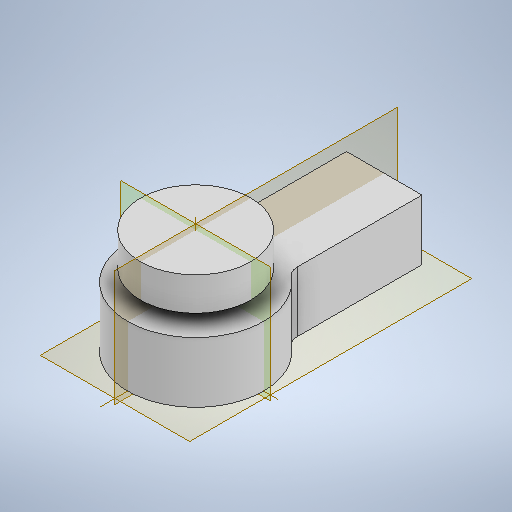
# Autodesk Inventor part: alternativeJoint2
Saved by Autodesk Inventor 2025.1 (Build 291241000, 241)
## iProperties
Created: 2024-11-07
Part Number: alternativeJoint2
Material: Generisch
Document SubType Name: Modeling
Designer: ZOMBULLI
Density: 1 g/cm^3
Appearance: Vorgabe
Author: ZOMBULLI
Autodesk Inventor part; units mm, degrees
sketch "Skizze1" plane through (0, 0, 0) normal (0, 0, 1) x (1, 0, 0)
  line L0 (5, 25) -> (-5, 25)
  line L1 (-5, 25) -> (-5, 9.3808)
  line L2 (5, 8.4853) -> (5, 25)
  arc A0 (-6.2308, 6.4944) -> (5.7273, 6.9425) centre (0, 0) ccw
  arc A1 (5, 8.4853) -> (5.7273, 6.9425) centre (7, 8.4853) ccw
  arc A2 (-6.2308, 6.4944) -> (-5, 9.3808) centre (-9, 9.3808) ccw
  line L3 (0, -25.0931) -> (0, 22.9698)
  line L4 (0, 35.0186) -> (0, -35.1118) projected
  point P0 (0, 0)
  point P1 (0, 0)
  point P2 (-5, 7.4833)
  point P3 (5, 7.4833)
  dimension "d1" = 18
  dimension "d2" = 5
  dimension "d3" = 2
  dimension "d4" = 4
  dimension "d5" = 10
  dimension "d6" = 5
  dimension "d7" = 0
  dimension "d8" = 25
  dimension "d9" = 0
  dimension "d10" = 0
  constraints: 8 end point, 8 point on circle, 4 tangent, 3 centre point, 2 point on line, 1 horizontal, 1 parallel, 1 perpendicular
  measures "d1" diameter of A0
  measures "d2" distance from line of A0.centre L2
  measures "d3" radius of A1
  measures "d4" radius of A2
  measures "d5" distance between parallel lines of L1 L2
  measures "d6" distance between parallel lines of L3 L2
  measures "d7" distance of A0.centre point (0, 0)
  measures "d8" distance from line of point (0, 0) L0
  measures "d9" distance between parallel lines of L4 L3
  measures "d10" distance of point (0, 0) point (0, 0)
extrude "Extrusion1" add sketch "Skizze1" along normal blind 8
sketch "Skizze3" plane through (0, 0, 0) normal (1, 0, 0) x (0, 1, 0)
  line L0 (6.9425, 8) -> (-9, 8) projected
  line L1 (0, 14) -> (4.9, 14)
  line L2 (4.9, 12.4) -> (4.9, 8)
  line L3 (4.9, 8) -> (0, 8)
  line L4 (0, 8) -> (0, 14)
  line L5 (4.9, 14) -> (7.3, 14)
  line L6 (7.3, 14) -> (7.3, 9.6)
  line L7 (7.3, 9.6) -> (6.1, 9.6)
  line L8 (6.1, 9.6) -> (6.1, 12.4)
  line L9 (6.1, 12.4) -> (4.9, 12.4)
  point P0 (0, 0)
  point P1 (6.4944, 8)
  point P2 (6.1, 11)
  point P3 (5.5, 12.4)
  point P4 (6.7, 9.6)
  dimension "d13" = 6
  dimension "d14" = 4.9
  dimension "d15" = 1.2
  dimension "d16" = 1.2
  dimension "d17" = 1.6
  dimension "d18" = 2.8
  constraints: 18 end point, 4 perpendicular, 3 midpoint, 2 horizontal, 2 parallel, 1 point on line, 1 vertical
  measures "d13" distance of L3.end L1.start
  measures "d14" distance between parallel lines of L2 L4
  measures "d15" distance of L6.end L7.end
  measures "d16" distance from line of point (6.1, 11) L2
  measures "d17" distance from line of L5 point (5.5, 12.4)
  measures "d18" distance from line of L9 point (6.7, 9.6)
revolve "Umdrehung1" add sketch "Skizze3" angle 360 about axis through (0, 0, 8) along (0, 0, 1)
